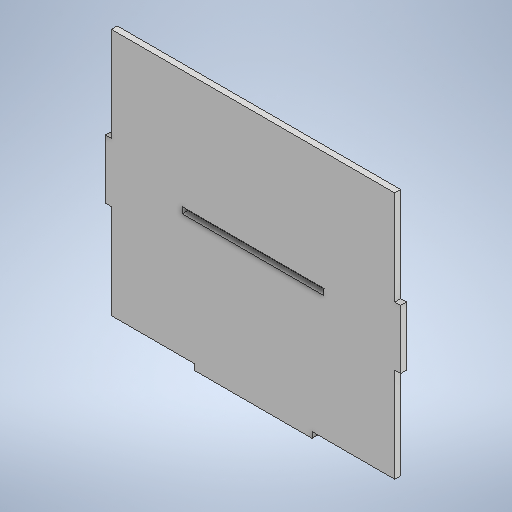
# Autodesk Inventor part: back
Saved by Autodesk Inventor 2025.3 (Build 293356030, 356C)
## iProperties
Created: 2026-06-26
Part Number: back
Material: Generic
Document SubType Name: Modeling
Designer: user
Density: 1 g/cm^3
Appearance: Default
Author: user
Autodesk Inventor part; units mm, degrees
ref_plane "YZ Plane" through (0, 0, 0) normal (1, 0, 0) x (0, 1, 0)
ref_plane "XZ Plane" through (0, 0, 0) normal (0, 1, 0) x (-1, 0, 0)
ref_plane "XY Plane" through (0, 0, 0) normal (0, 0, 1) x (1, 0, 0)
sketch "Sketch1" plane through (0, 0, 0) normal (0, 0, 1) x (1, 0, 0)
  line L0 (0, 0) -> (240, 0)
  line L1 (240, 0) -> (240, 210)
  line L2 (240, 210) -> (0, 210)
  line L3 (0, 210) -> (0, 0)
  line L4 (0, 80) -> (-5, 80)
  line L5 (-5, 80) -> (-5, 130)
  line L6 (-5, 130) -> (0, 130)
  line L7 (0, 130) -> (0, 80)
  line L8 (120, 0) -> (120, 210) construction
  line L9 (240, 80) -> (245, 80)
  line L10 (245, 80) -> (245, 130)
  line L11 (245, 130) -> (240, 130)
  line L12 (240, 130) -> (240, 80)
  line L13 (60, 104.7) -> (180, 104.7)
  line L14 (180, 104.7) -> (180, 110)
  line L15 (180, 110) -> (60, 110)
  line L16 (60, 110) -> (60, 104.7)
  line L17 (70, 0) -> (170, 0)
  line L18 (170, 0) -> (170, -5)
  line L19 (170, -5) -> (70, -5)
  line L20 (70, -5) -> (70, 0)
  point P0 (240, 80)
  point P1 (170, 0)
  dimension "d0" = 240
  dimension "d1" = 210
  dimension "d2" = 5
  dimension "d3" = 50
  dimension "d6" = 120
  dimension "d7" = 5.3
  dimension "d10" = 100
  dimension "d11" = 5
  dimension "d12" = 50
  constraints: 42 end point, 8 parallel, 4 horizontal, 4 perpendicular, 4 symmetric about line, 2 midpoint, 2 point on line
  measures "d0" distance of L2.end L1.end
  measures "d1" distance of L1.end L0.end
  measures "d2" distance of L5.end L6.end
  measures "d3" distance of L4.end L5.end
  measures "d6" distance of L15.end L14.end
  measures "d7" distance of L14.end L13.end
  measures "d10" distance of L18.end L19.end
  measures "d11" distance of L17.end L18.end
  measures "d12" distance between parallel lines of L18 L8
extrude "Extrusion1" add sketch "Sketch1" along normal blind 5
body "Solid1"
